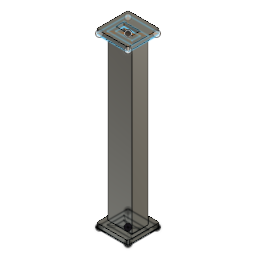
WaveguideKu (Autodesk Fusion 360 design; units mm, degrees)
Autodesk Fusion 360 part; units mm, degrees
sketch "Sketch1" plane through (0, 0, 0) normal (0, 0, 1) x (1, 0, 0)
  line L0 (17.05, 19.05) -> (-17.05, 19.05)
  line L1 (-19.05, 17.05) -> (-19.05, -17.05)
  line L2 (-17.05, -19.05) -> (17.05, -19.05)
  line L3 (19.05, -17.05) -> (19.05, 17.05)
  line L4 (19.05, 19.05) -> (-19.05, -19.05) construction
  line L5 (-19.05, 19.05) -> (19.05, -19.05) construction
  arc A0 (-17.05, 19.05) -> (-19.05, 17.05) centre (-17.05, 17.05) ccw
  arc A1 (19.05, 17.05) -> (17.05, 19.05) centre (17.05, 17.05) ccw
  arc A2 (17.05, -19.05) -> (19.05, -17.05) centre (17.05, -17.05) ccw
  arc A3 (-19.05, -17.05) -> (-17.05, -19.05) centre (-17.05, -17.05) ccw
  line L6 (9.525, 4.765) -> (-9.525, 4.765)
  line L7 (-9.525, 4.765) -> (-9.525, -4.765)
  line L8 (-9.525, -4.765) -> (9.525, -4.765)
  line L9 (9.525, -4.765) -> (9.525, 4.765)
  line L10 (9.525, 4.765) -> (-9.525, -4.765) construction
  line L11 (-9.525, 4.765) -> (9.525, -4.765) construction
  line L12 (14.525, 9.765) -> (-14.525, 9.765)
  line L13 (-14.525, 9.765) -> (-14.525, -9.765)
  line L14 (-14.525, -9.765) -> (14.525, -9.765)
  line L15 (14.525, -9.765) -> (14.525, 9.765)
  line L16 (14.525, 9.765) -> (-14.525, -9.765) construction
  line L17 (-14.525, 9.765) -> (14.525, -9.765) construction
  line L18 (19.05, 19.05, 200) -> (-19.05, -19.05, 200) construction
  arc A4 through (-19.05, -17.05, 200) (-18.4642, -18.4642, 200) (-17.05, -19.05, 200)
  line L19 (-17.05, -19.05, 200) -> (17.05, -19.05, 200)
  line L20 (9.525, 4.765, 200) -> (-9.525, -4.765, 200) construction
  arc A5 through (-17.05, 19.05, 200) (-18.4642, 18.4642, 200) (-19.05, 17.05, 200)
  line L21 (-9.525, -4.765, 200) -> (9.525, -4.765, 200)
  line L22 (-14.525, 9.765, 200) -> (14.525, -9.765, 200) construction
  line L23 (-19.05, 17.05, 200) -> (-19.05, -17.05, 200)
  line L24 (17.05, 19.05, 200) -> (-17.05, 19.05, 200)
  line L25 (-14.525, 9.765, 200) -> (-14.525, -9.765, 200)
  line L26 (-19.05, 19.05, 200) -> (19.05, -19.05, 200) construction
  line L27 (9.525, -4.765, 200) -> (9.525, 4.765, 200)
  arc A6 through (19.05, 17.05, 200) (18.4642, 18.4642, 200) (17.05, 19.05, 200)
  line L28 (19.05, -17.05, 200) -> (19.05, 17.05, 200)
  arc A7 through (17.05, -19.05, 200) (18.4642, -18.4642, 200) (19.05, -17.05, 200)
  line L29 (14.525, 9.765, 200) -> (-14.525, 9.765, 200)
  line L30 (9.525, 4.765, 200) -> (-9.525, 4.765, 200)
  line L31 (-9.525, 4.765, 200) -> (-9.525, -4.765, 200)
  line L32 (14.525, -9.765, 200) -> (14.525, 9.765, 200)
  line L33 (14.525, 9.765, 200) -> (-14.525, -9.765, 200) construction
  line L34 (-14.525, -9.765, 200) -> (14.525, -9.765, 200)
  line L35 (-9.525, 4.765, 200) -> (9.525, -4.765, 200) construction
  dimension "d9" = 38.1
  dimension "d10" = 38.1
  dimension "d11" = 2
  dimension "d12" = 2
  dimension "d13" = 2
  dimension "d14" = 2
  dimension "d15" = 19.05
  dimension "d16" = 9.53
  dimension "d17" = 29.05
  dimension "d18" = 19.53
  dimension "d19" = 38.1
  dimension "d20" = 38.1
  dimension "d21" = 2
  dimension "d22" = 2
  dimension "d23" = 2
  dimension "d24" = 2
  dimension "d25" = 19.05
  dimension "d26" = 9.53
  dimension "d27" = 29.05
  dimension "d28" = 19.53
  constraint horizontal L0
  constraint perpendicular L0 L1
  constraint parallel L0 L2
  constraint parallel L1 L3
  constraint coincident L4 origin
  constraint coincident L5 origin
  constraint coincident L5.start L1
  constraint coincident L5.start L0
  constraint tangent L1 A0
  constraint tangent L0 A0
  constraint coincident L4.start L0
  constraint coincident L4.start L3
  constraint tangent L0 A1
  constraint tangent L3 A1
  constraint coincident L5.end L3
  constraint coincident L5.end L2
  constraint tangent L3 A2
  constraint tangent L2 A2
  constraint coincident L4.end L1
  constraint coincident L4.end L2
  constraint tangent L1 A3
  constraint tangent L2 A3
  constraint horizontal L6
  constraint perpendicular L6 L7
  constraint parallel L6 L8
  constraint parallel L7 L9
  constraint coincident L10 origin
  constraint coincident L11 origin
  constraint horizontal L12
  constraint perpendicular L12 L13
  constraint parallel L12 L14
  constraint parallel L13 L15
  constraint coincident L16 origin
  constraint coincident L17 origin
  measures "d9" distance of L4.end L5.end
  measures "d10" distance of L5.start L4.end
  measures "d11" radius of A0
  measures "d12" radius of A1
  measures "d13" radius of A2
  measures "d14" radius of A3
  measures "d15" distance of L7.end L8.end
  measures "d16" distance of L6.end L7.end
  measures "d17" distance of L13.end L14.end
  measures "d18" distance of L12.end L13.end
  measures "d19" distance of L5.end L4.end
  measures "d20" distance of L5.start L4.end
  measures "d25" distance of L7.end L8.end
  measures "d26" distance of L7.end L6.end
  measures "d27" distance of L14.end L13.end
  measures "d28" distance of L12.end L13.end
extrude "Extrude1" add sketch "Sketch1" along normal blind 5 contours L0 L1 L2 L3 A0 A1 A2 A3 makes body 1
extrude "Extrude2" add sketch "Sketch1" along normal blind 5 separate body contours A4 L19 A5 L23 L24 A6 L28 A7 in plane through (0, 0, 200) normal (0, 0, 1) makes body 2
extrude "Extrude3" add sketch "Sketch1" along normal blind 200 contours L12 L13 L14 L15 bodies 1 2
extrude "Extrude4" add sketch "Sketch1" along normal blind 5 contours L25 L29 L32 L34 in plane through (0, 0, 200) normal (0, 0, 1) bodies 1
equation "innerWidth = 19.05 mm"
equation "innerHeight = 9.53 mm"
equation "flangeWidth = 38.10 mm"
equation "flangeHeight = 38.10 mm"
equation "holeDia = 4.1 mm"
equation "offsetWidth = 29.05 mm"
equation "offsetHeight = 19.53 mm"
equation "Length = 200.0 mm"
equation "d9 = flangeWidth"
equation "d10 = flangeHeight"
equation "d15 = innerWidth"
equation "d16 = innerHeight"
equation "d17 = offsetWidth"
equation "d18 = offsetHeight"
equation "d19 = flangeWidth"
equation "d20 = flangeHeight"
equation "d25 = innerWidth"
equation "d26 = innerHeight"
equation "d27 = offsetWidth"
equation "d28 = offsetHeight"
